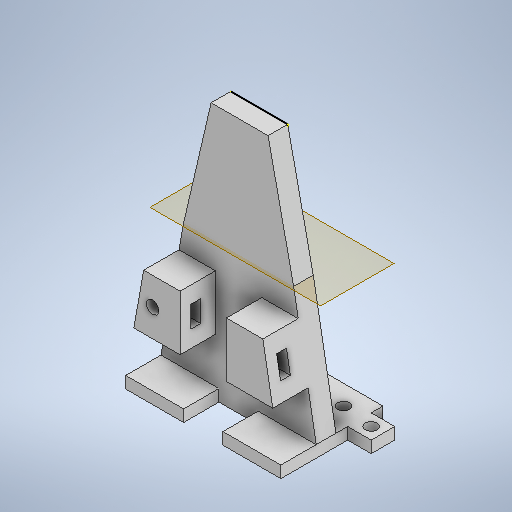
# Autodesk Inventor part: plate
Saved by Autodesk Inventor 2025 (Build 290162000, 162)
## iProperties
Created: 2025-06-05
Part Number: plate
Material: Generic
Document SubType Name: Modeling
Designer: omiye
Density: 1 g/cm^3
Appearance: Default
Author: omiye
Autodesk Inventor part; units mm, degrees
ref_plane "YZ Plane" through (0, 0, 0) normal (1, 0, 0) x (0, 1, 0)
ref_plane "XZ Plane" through (0, 0, 0) normal (0, 1, 0) x (-1, 0, 0)
ref_plane "XY Plane" through (0, 0, 0) normal (0, 0, 1) x (1, 0, 0)
sketch "Sketch1" plane through (0, 0, 0) normal (0, 1, 0) x (-1, 0, 0)
  line L0 (-50, 15) -> (50, 15)
  line L1 (50, 15) -> (50, -15)
  line L2 (50, -15) -> (-50, -15)
  line L3 (-50, -15) -> (-50, 15)
  line L4 (-50, 15) -> (50, -15) construction
  line L5 (50, 15) -> (-50, -15) construction
  point P0 (0, 0)
  dimension "d0" = 100
  dimension "d1" = 30
  constraints: 12 end point, 2 midpoint, 2 parallel, 1 horizontal, 1 perpendicular
  measures "d0" distance of L1.end L2.end
  measures "d1" distance of L0.end L1.end
extrude "Extrusion1" add sketch "Sketch1" along normal blind 3
sketch "Sketch2" plane through (0, 3, 0) normal (0, 1, 0) x (1, 0, 0)
  line L0 (25, -5) -> (-25, -5)
  line L1 (-25, -5) -> (-25, 5)
  line L2 (-25, 5) -> (25, 5)
  line L3 (25, 5) -> (25, -5)
  line L4 (25, -5) -> (-25, 5) construction
  line L5 (-25, -5) -> (25, 5) construction
  line L6 (50, 15) -> (-50, 15) projected
  line L7 (50, -15) -> (-50, -15)
  line L8 (-50, -15) -> (-50, 15)
  line L9 (-50, 15) -> (50, 15)
  line L10 (50, 15) -> (50, -15)
  line L11 (50, -15) -> (-50, 15) construction
  line L12 (-50, -15) -> (50, 15) construction
  point P0 (0, 0)
  dimension "d4" = 50
  dimension "d5" = 10
  constraints: 24 end point, 4 midpoint, 4 parallel, 2 horizontal, 2 perpendicular
  measures "d4" distance of L1.end L2.end
  measures "d5" distance of L0.end L1.end
extrude "Extrusion2" cut sketch "Sketch2" against normal blind 3
sketch "Sketch3" plane through (0, 0, 0) normal (0, -1, 0) x (1, 0, 0)
  line L0 (0, 0) -> (5, 0)
  line L1 (5, 0) -> (-5, 0)
  circle A0 centre (-5, 0) radius 1.1
  circle A1 centre (5, 0) radius 1.1
  line L2 (5, 0) -> (14.75, 0)
  line L3 (-5, 0) -> (-14.75, 0)
  circle A2 centre (14.75, 0) radius 1.1
  circle A3 centre (-14.75, 0) radius 1.1
  dimension "d8" = 5
  dimension "d9" = 10
  dimension "d10" = 2.2
  dimension "d11" = 2.2
  dimension "d12" = 9.75
  dimension "d13" = 9.75
  dimension "d14" = 2.2
  dimension "d15" = 2.2
  constraints: 8 end point, 4 centre point, 4 coincident, 2 horizontal, 2 point on line
  measures "d8" distance of L0.start L0.end
  measures "d9" distance of L0.end L1.end
  measures "d10" diameter of A0
  measures "d11" diameter of A1
  measures "d12" distance of L2.start L2.end
  measures "d13" distance of L3.start L3.end
  measures "d14" diameter of A2
  measures "d15" diameter of A3
extrude "Extrusion3" cut sketch "Sketch3" against normal blind 3.95
sketch "Sketch4" plane through (0, 3, 0) normal (0, 1, 0) x (1, 0, 0)
  circle A0 centre (-14.75, 0) radius 1.1 projected
  line L0 (-14.75, 0) -> (-19.75, 0)
  line L1 (-19.75, 0) -> (-19.75, 5)
  line L2 (25, 5) -> (-25, 5) projected
  line L3 (-19.75, 0) -> (-19.75, -5)
  line L4 (-25, -5) -> (25, -5) projected
  circle A1 centre (14.75, 0) radius 1.1 projected
  line L5 (14.75, 0) -> (19.75, 0)
  line L6 (19.75, 0) -> (19.75, 5.4669)
  line L7 (19.75, 5.4669) -> (19.75, -5)
  line L8 (-25, 5) -> (-19.75, 5)
  line L9 (-19.75, 5) -> (-19.75, -5)
  line L10 (-19.75, -5) -> (-25, -5)
  line L11 (-25, -5) -> (-25, 5)
  line L12 (19.75, -5) -> (25, -5)
  line L13 (25, -5) -> (25, 5)
  line L14 (25, 5) -> (19.75, 5)
  line L15 (19.75, 5) -> (19.75, -5)
  point P0 (0, 0)
  dimension "d18" = 5
  dimension "d19" = 5
  constraints: 28 end point, 5 point on line, 4 parallel, 4 perpendicular, 3 horizontal
  measures "d18" distance of L0.start L0.end
  measures "d19" distance of L5.start L5.end
extrude "Extrusion4" cut sketch "Sketch4" against normal blind 3.95 contours L3 L4 L11 L2 L1 | L2 L13 L4 L7 L6
sketch "Sketch5" plane through (0, 3, 0) normal (0, 1, 0) x (1, 0, 0)
  circle A0 centre (-14.75, 0) radius 1.1 projected
  line L0 (-14.75, 0) -> (-14.75, -12)
  line L1 (-19.75, -5) -> (19.75, -5) projected
  line L2 (-14.75, 0) -> (-2.75, 0) construction
  line L3 (-14.75, -12) -> (14.75, -12)
  circle A1 centre (14.75, 0) radius 1.1 projected
  line L4 (14.75, -12) -> (14.75, 0)
  line L5 (14.75, 0) -> (-14.75, 0)
  line L6 (-14.75, -12) -> (14.75, -12)
  line L7 (14.75, -12) -> (14.75, -10)
  line L8 (14.75, -10) -> (-14.75, -10)
  line L9 (-14.75, -10) -> (-14.75, -12)
  line L10 (2.5, -24) -> (-2.5, -24)
  line L11 (-2.5, -24) -> (-2.5, 0)
  line L12 (-2.5, 0) -> (2.5, 0)
  line L13 (2.5, 0) -> (2.5, -24)
  line L14 (2.5, -24) -> (-2.5, 0) construction
  line L15 (-2.5, -24) -> (2.5, 0) construction
  line L16 (-14.75, -12) -> (-19.75, -12)
  line L17 (-19.75, -12) -> (-19.75, -5)
  line L18 (-19.75, -5) -> (-14.75, -5)
  line L19 (-14.75, -5) -> (-14.75, -12)
  line L20 (14.75, -12) -> (19.75, -12)
  line L21 (19.75, -12) -> (19.75, -5)
  line L22 (19.75, -5) -> (14.75, -5)
  line L23 (14.75, -5) -> (14.75, -12)
  point P0 (0, 0)
  point P1 (0, -12)
  point P2 (2.5, -5)
  point P3 (2.5, -10)
  point P4 (-2.5, -10)
  point P5 (-2.5, -5)
  dimension "d22" = 12
  dimension "d23" = 90
  dimension "d24" = 2
  dimension "d25" = 5
  constraints: 46 end point, 9 perpendicular, 8 parallel, 4 horizontal, 3 midpoint, 1 point on line
  measures "d22" distance of L0.start L0.end
  measures "d23" angle of L0 L2
  measures "d24" distance of L7.end L6.end
  measures "d25" distance of L10.start L10.end
extrude "Extrusion5" add sketch "Sketch5" against normal up to surface (3 mm away) contours L1 L11 L8 L0 | L0 L16 L17 L1 | L8 L11 L3 L0 | L1 L4 L8 L13 | L8 L13 L3 L11 | L1 L21 L20 L4 | L8 L4 L3 L13
sketch "Sketch6" plane through (0, 3, 0) normal (0, 1, 0) x (1, 0, 0)
  line L0 (-19.75, -12) -> (-19.75, 5) projected
  line L1 (19.75, 5) -> (19.75, -12) projected
  line L2 (-19.75, -12) -> (19.75, -12)
  line L3 (19.75, -12) -> (19.75, -10)
  line L4 (19.75, -10) -> (-19.75, -10)
  line L5 (-19.75, -10) -> (-19.75, -12)
  point P0 (0, 0)
  dimension "d28" = 2
  constraints: 8 end point, 2 parallel, 1 horizontal, 1 perpendicular, 1 point on line
  measures "d28" distance of L3.end L2.end
ref_plane "Work Plane2" through (0, 35, 0) normal (0, 1, 0) x (1, 0, 0)
sketch "Sketch10" plane through (0, 35, 0) normal (0, 1, 0) x (1, 0, 0)
  line L0 (-19.75, -12) -> (19.75, -12) projected
  line L1 (0, -12) -> (-14, -12)
  line L2 (-14, -12) -> (14, -12)
  line L3 (14, -12) -> (14, -10)
  line L4 (14, -10) -> (-14, -10)
  line L5 (-14, -10) -> (-14, -12)
  point P0 (0, 0)
  dimension "d43" = 14
  dimension "d44" = 28
  dimension "d45" = 2
  constraints: 10 end point, 2 perpendicular, 2 point on line, 1 midpoint, 1 parallel
  measures "d43" distance of L1.start L1.end
  measures "d44" distance of L1.end L2.end
  measures "d45" distance of L2.end L3.end
loft "Loft2" add profiles "Sketch10", "Sketch6"
sketch "Sketch11" plane through (-14, 35, 12) normal (0, 1, 0) x (1, 0, 0)
  line L0 (33.75, 0) -> (-5.75, 0) projected
  line L1 (14, 0) -> (7, 0)
  line L2 (7, 0) -> (21, 0)
  line L3 (28, 2) -> (0, 2) projected
  line L4 (7, 0) -> (21.5, 0)
  line L5 (21.5, 0) -> (21.5, 2)
  line L6 (21.5, 2) -> (7, 2)
  line L7 (7, 2) -> (7, 0)
  point P0 (14, 12)
  point P1 (7, 2)
  point P2 (21.5, 0)
  dimension "d50" = 7
  dimension "d51" = 14
  constraints: 12 end point, 3 point on line, 2 parallel, 1 horizontal, 1 midpoint, 1 perpendicular
  measures "d50" distance of L1.start L1.end
  measures "d51" distance of L1.end L2.end
extrude "Extrusion7" add sketch "Sketch11" along normal blind 30
sketch "Sketch12" plane through (2.5, 0, 10) normal (0, 0, -1) x (-1, 0, 0)
  line L0 (2.5, 35) -> (2.5, 3)
  line L1 (5, 3) -> (0, 3) projected
  circle A0 centre (2.5, 19) radius 12.35
  point P0 (2.5, 0)
  dimension "d54" = 24.7
  constraints: 2 end point, 2 midpoint, 1 centre point
  measures "d54" diameter of A0
sketch "Sketch13" plane through (2.5, 0, 10) normal (0, 0, -1) x (-1, 0, 0)
  line L0 (16.5, 35) -> (9.5, 35) projected
  line L1 (16.5, 35) -> (9.5, 35)
  line L2 (-5, 65) -> (9.5, 65) projected
  line L3 (9.5, 35) -> (9.5, 65)
  line L4 (-5, 35) -> (-5, 65) projected
  line L5 (9.5, 65) -> (-5, 65)
  line L6 (-5, 65) -> (-5, 35)
  line L7 (-11.5, 35) -> (-5, 35) projected
  line L8 (-5, 35) -> (-11.5, 35)
  line L9 (-17.25, 3) -> (-17.25, 0) projected
  line L10 (-11.5, 35) -> (-17.25, 3)
  line L11 (16.5, 35) -> (22.25, 3) projected
  line L12 (-17.25, 3) -> (22.25, 3)
  line L13 (22.25, 3) -> (16.5, 35)
  circle A0 centre (2.5, 19) radius 12.35
  line L14 (9.5, 35) -> (-5, 35)
  point P0 (2.5, 0)
  dimension "d55" = 24.7
  constraints: 18 end point, 3 perpendicular, 2 collinear, 2 horizontal, 1 centre point, 1 parallel
  measures "d55" diameter of A0
extrude "Extrusion8" add sketch "Sketch13" along normal blind 3
extrude "Extrusion9" cut sketch "Sketch12" against normal blind 0.5
sketch "Sketch14" plane through (-2.5, 3, 5) normal (0, 0, 1) x (1, 0, 0)
  line L0 (0, 0) -> (5, 0) projected
  line L1 (0, 0) -> (0, -3) projected
  line L2 (5, 0) -> (0, 0)
  line L3 (0, 0) -> (0, -3)
  line L4 (0, -3) -> (5, -3)
  line L5 (5, -3) -> (5, 0)
  point P0 (2.5, -3)
  constraints: 8 end point, 2 parallel, 1 horizontal, 1 perpendicular
extrude "Extrusion10" cut sketch "Sketch14" against normal blind 2.5
sketch "Sketch15" plane through (-19.75, 0, 12) normal (0, 0, 1) x (1, 0, 0)
  line L0 (0, 0) -> (0, 3) projected
  line L1 (0, 0) -> (39.5, 0) projected
  line L2 (0, 3) -> (39.5, 3)
  line L3 (39.5, 3) -> (39.5, 0)
  line L4 (39.5, 0) -> (0, 0)
  line L5 (0, 0) -> (0, 3)
  point P0 (19.75, 0)
  constraints: 8 end point, 2 parallel, 1 horizontal, 1 perpendicular
extrude "Extrusion11" add sketch "Sketch15" along normal blind 9
sketch "Sketch16" plane through (-7, 65, 12) normal (0, 0, 1) x (1, 0, 0)
  line L0 (-12.75, -62) -> (26.75, -62) projected
  line L1 (7, -62) -> (7, -50.5)
  line L2 (7, -50.5) -> (1.1, -50.5)
  line L3 (1.1, -50.5) -> (7, -50.5)
  line L4 (7, -50.5) -> (12.9, -50.5)
  line L5 (12.9, -50.5) -> (22.9, -50.5)
  line L6 (22.9, -50.5) -> (1.1, -50.5)
  line L7 (1.1, -50.5) -> (-8.9, -50.5)
  line L8 (-8.9, -50.5) -> (-8.9, -36.5)
  line L9 (-8.9, -36.5) -> (1.1, -36.5)
  line L10 (1.1, -36.5) -> (1.1, -50.5)
  line L11 (12.9, -50.5) -> (12.9, -36.5)
  line L12 (12.9, -36.5) -> (22.9, -36.5)
  line L13 (22.9, -36.5) -> (22.9, -50.5)
  line L14 (1.1, -50.5) -> (-1.9, -50.5)
  line L15 (-1.9, -50.5) -> (-1.9, -36.5)
  line L16 (-1.9, -36.5) -> (1.1, -36.5)
  line L17 (1.1, -36.5) -> (1.1, -50.5)
  line L18 (12.9, -50.5) -> (15.9, -50.5)
  line L19 (15.9, -50.5) -> (15.9, -36.5)
  line L20 (15.9, -36.5) -> (12.9, -36.5)
  line L21 (12.9, -36.5) -> (12.9, -50.5)
  point P0 (7, -65)
  dimension "d64" = 11.5
  dimension "d65" = 5.9
  dimension "d66" = 5.9
  dimension "d67" = 10
  dimension "d68" = 10
  dimension "d69" = 14
  dimension "d70" = 3
  dimension "d71" = 3
  constraints: 42 end point, 5 parallel, 4 horizontal, 4 perpendicular, 4 point on line, 4 vertical, 2 collinear, 1 midpoint
  measures "d64" distance of L1.start L1.end
  measures "d65" distance of L1.end L2.end
  measures "d66" distance of L1.end L4.end
  measures "d67" distance of L4.end L5.end
  measures "d68" distance of L2.end L7.end
  measures "d69" distance of L7.end L8.end
  measures "d70" distance of L15.end L16.end
  measures "d71" distance of L20.end L19.end
extrude "Extrusion12" add sketch "Sketch16" along normal up to surface (9 mm away) contours L11 L12 L19 L5 | L7 L15 L9 L10
sketch "Sketch17" plane through (-8.9, 14.5, 21) normal (0, 0, 1) x (1, 0, 0)
  line L0 (0, 14) -> (3, 14) projected
  line L1 (0, 14) -> (-8, 14)
  line L2 (-8, 14) -> (-8, 0)
  line L3 (-8, 0) -> (0, 0)
  line L4 (0, 0) -> (0, 14)
  line L5 (17.8, 14) -> (17.8, 0) projected
  line L6 (17.8, 14) -> (25.8, 14)
  line L7 (25.8, 14) -> (25.8, 0)
  line L8 (25.8, 0) -> (17.8, 0)
  line L9 (17.8, 0) -> (17.8, 14)
  line L10 (-8, 7) -> (-4, 7)
  circle A0 centre (-4, 7) radius 1.6
  line L11 (25.8, 0) -> (21.8, 0)
  line L12 (25.8, 7) -> (21.8, 7)
  circle A1 centre (21.8, 7) radius 1.6
  point P0 (8.9, -14.5)
  dimension "d74" = 8
  dimension "d75" = 8
  dimension "d76" = 3.2
  dimension "d77" = 3.2
  constraints: 22 end point, 4 horizontal, 4 parallel, 3 midpoint, 2 centre point, 2 coincident, 2 perpendicular, 1 point on line
  measures "d74" distance of L3.end L2.end
  measures "d75" distance of L7.end L8.end
  measures "d76" diameter of A0
  measures "d77" diameter of A1
extrude "Extrusion13" add sketch "Sketch17" against normal blind 3
sketch "Sketch18" plane through (-19.75, 0, -5) normal (-1, 0, 0) x (0, 0, 1)
  line L0 (0, 0) -> (0, 3) projected
  line L1 (12, 35) -> (12, 3) projected
  line L2 (0, 0) -> (12, 0)
  line L3 (12, 0) -> (12, 3)
  line L4 (12, 3) -> (0, 3)
  line L5 (0, 3) -> (0, 0)
  line L6 (12, 3) -> (0, 3) projected
  line L7 (5, 0) -> (9, 0)
  line L8 (9, 0) -> (9, 3)
  line L9 (9, 3) -> (5, 3)
  line L10 (5, 3) -> (5, 0)
  line L11 (5, 0) -> (3, 0)
  line L12 (3, 0) -> (3, 3)
  line L13 (3, 3) -> (5, 3)
  line L14 (5, 3) -> (5, 0)
  point P0 (3, 3)
  point P1 (3, 0)
  dimension "d80" = 4
  dimension "d81" = 2
  constraints: 24 end point, 6 parallel, 3 horizontal, 3 perpendicular, 2 point on line
  measures "d80" distance of L9.end L8.end
  measures "d81" distance of L12.end L13.end
extrude "Extrusion14" add sketch "Sketch18" along normal blind 6 contours L12 L4 L10 L2 | L10 L4 L8 L2
sketch "Sketch19" plane through (19.75, 0, -5) normal (1, 0, 0) x (0, 0, -1)
  line L0 (-9, 3) -> (-3, 3) projected
  line L1 (-5, 0) -> (-9, 0)
  line L2 (-9, 0) -> (-9, 3)
  line L3 (-9, 3) -> (-5, 3)
  line L4 (-5, 3) -> (-5, 0)
  line L5 (-5, 0) -> (-3, 0)
  line L6 (-3, 0) -> (-3, 3)
  line L7 (-3, 3) -> (-5, 3)
  line L8 (-5, 3) -> (-5, 0)
  dimension "d84" = 4
  dimension "d85" = 2
  constraints: 16 end point, 4 parallel, 2 horizontal, 2 perpendicular, 1 point on line
  measures "d84" distance of L0.start L3.end
  measures "d85" distance of L7.end L6.end
extrude "Extrusion15" add sketch "Sketch19" along normal blind 6
sketch "Sketch20" plane through (0, 3, 0) normal (0, 1, 0) x (1, 0, 0)
  line L0 (25.75, -4) -> (25.75, 2) projected
  line L1 (25.75, -1) -> (22.75, -1)
  circle A0 centre (22.75, -1) radius 1.525
  line L2 (-25.75, -4) -> (-25.75, 2) projected
  line L3 (-25.75, -1) -> (-22.75, -1)
  circle A1 centre (-22.75, -1) radius 1.525
  point P0 (0, 0)
  dimension "d88" = 3
  dimension "d89" = 3.05
  dimension "d90" = 3
  dimension "d91" = 3.05
  constraints: 4 end point, 2 centre point, 2 coincident, 2 horizontal, 2 midpoint
  measures "d88" distance of L1.start L1.end
  measures "d89" diameter of A0
  measures "d90" distance of L3.start L3.end
  measures "d91" diameter of A1
extrude "Extrusion16" cut sketch "Sketch20" against normal blind 6
sketch "Sketch21" plane through (2.5, 0, 7) normal (0, 0, -1) x (-1, 0, 0)
  line L0 (9.5, 35) -> (9.5, 65) projected
  line L1 (-5, 35) -> (-5, 65) projected
  line L2 (9.5, 65) -> (-5, 65)
  line L3 (-5, 65) -> (-5, 35)
  line L4 (-5, 35) -> (9.5, 35)
  line L5 (9.5, 35) -> (9.5, 65)
  point P0 (2.5, 0)
  constraints: 8 end point, 2 parallel, 1 horizontal, 1 perpendicular
sketch "Sketch22" plane through (2.5, 0, 7) normal (0, 0, -1) x (-1, 0, 0)
  line L0 (16.5, 35) -> (9.5, 35) projected
  line L1 (9.5, 35) -> (9.5, 65) projected
  line L2 (16.5, 35) -> (9.5, 65)
  line L3 (-5, 35) -> (-5, 65) projected
  line L4 (9.5, 65) -> (-5, 65)
  line L5 (-11.5, 35) -> (-17.25, 3) projected
  line L6 (-5, 65) -> (-11.5, 35)
  line L7 (-5, 35) -> (-11.5, 35) projected
  line L8 (-5, 35) -> (-11.5, 35)
  point P0 (2.5, 0)
  constraints: 8 end point, 1 collinear, 1 perpendicular
extrude "Extrusion17" add sketch "Sketch22" against normal up to surface (5 mm away)
sketch "Sketch23" plane through (0, 3, 0) normal (0, 1, 0) x (1, 0, 0)
  circle A0 centre (-14.75, 0) radius 1.1 projected
  circle A1 centre (-14.75, 0) radius 1.5
  circle A2 centre (-5, 0) radius 1.1 projected
  circle A3 centre (-5, 0) radius 1.5
  circle A4 centre (5, 0) radius 1.1 projected
  circle A5 centre (5, 0) radius 1.5
  circle A6 centre (14.75, 0) radius 1.1 projected
  circle A7 centre (14.75, 0) radius 1.5
  point P0 (0, 0)
  dimension "d96" = 3
  dimension "d97" = 3
  dimension "d98" = 3
  dimension "d99" = 3
  constraints: 4 centre point, 4 coincident
  measures "d96" diameter of A1
  measures "d97" diameter of A3
  measures "d98" diameter of A5
  measures "d99" diameter of A7
extrude "Extrusion18" cut sketch "Sketch23" against normal blind 10 contours A0 | A1 | A3 | A4 | A5 | A6 | A7
sketch "Sketch24" plane through (-19.75, 3, 12) normal (0, 0, 1) x (1, 0, 0)
  line L0 (10.85, 11.5) -> (2.85, 11.5) projected
  line L1 (2.85, 11.5) -> (2.0664, 11.5)
  line L2 (0, 0) -> (5.75, 32) projected
  line L3 (2.0664, 11.5) -> (4.582, 25.5)
  line L4 (10.85, 25.5) -> (13.85, 25.5) projected
  line L5 (13.85, 25.5) -> (4.582, 25.5)
  line L6 (13.85, 25.5) -> (13.85, 11.5)
  line L7 (13.85, 11.5) -> (2.0664, 11.5)
  circle A0 centre (6.85, 18.5) radius 1.6 projected
  circle A1 centre (6.85, 18.5) radius 1.6
  line L8 (13.85, 11.5) -> (13.85, 25.5)
  line L9 (33.75, 32) -> (39.5, 0) projected
  line L10 (34.918, 25.5) -> (37.4336, 11.5)
  line L11 (25.65, 11.5) -> (36.65, 11.5) projected
  line L12 (25.65, 11.5) -> (37.4336, 11.5)
  line L13 (25.65, 25.5) -> (28.65, 25.5) projected
  line L14 (25.65, 11.5) -> (25.65, 25.5)
  line L15 (25.65, 25.5) -> (34.918, 25.5)
  circle A2 centre (32.65, 18.5) radius 1.6 projected
  circle A3 centre (32.65, 18.5) radius 1.6
  point P0 (19.75, -3)
  dimension "d102" = 3.2
  constraints: 20 end point, 4 point on line, 3 collinear, 3 perpendicular, 2 centre point, 2 coincident, 1 horizontal, 1 vertical
  measures "d102" diameter of A1
extrude "Extrusion19" add sketch "Sketch24" along normal up to surface (9 mm away) contours L0 L1 L2 L5 L4 L6 L7 | L9 L12 L11 L14 L13 L15 | A2
sketch "Sketch25" plane through (-17.6836, 14.5, 21) normal (0, 0, 1) x (1, 0, 0)
  line L0 (0.7836, 14) -> (2.5156, 14) projected
  line L1 (2.5156, 14) -> (0.7836, 4.3609) projected
  line L2 (2.5156, 14) -> (0.7836, 4.3609)
  line L3 (0.7836, 4.3609) -> (0.7836, 14) projected
  line L4 (0.7836, 4.3609) -> (0.7836, 14)
  line L5 (0.7836, 14) -> (2.5156, 14)
  line L6 (34.5836, 4.3609) -> (32.8516, 14) projected
  line L7 (32.8516, 14) -> (34.5836, 4.3609)
  line L8 (34.5836, 4.3609) -> (34.5836, 14) projected
  line L9 (34.5836, 4.3609) -> (34.5836, 14)
  line L10 (34.5836, 14) -> (32.8516, 14)
  point P0 (17.6836, -14.5)
  constraints: 12 end point, 4 collinear, 2 perpendicular
extrude "Extrusion20" cut sketch "Sketch25" against normal blind 10
sketch "Sketch26" plane through (-19.75, 3, 7) normal (-1, 0, 0) x (0, 0, 1)
  line L0 (14, 11.5) -> (14, 25.5) projected
  line L1 (14, 18.5) -> (10, 18.5)
  line L2 (11.25, 15.75) -> (11.25, 21.25)
  line L3 (11.25, 21.25) -> (8.75, 21.25)
  line L4 (8.75, 21.25) -> (8.75, 15.75)
  line L5 (8.75, 15.75) -> (11.25, 15.75)
  line L6 (11.25, 15.75) -> (8.75, 21.25) construction
  line L7 (11.25, 21.25) -> (8.75, 15.75) construction
  line L8 (5, 16.9) -> (14, 16.9) projected
  line L9 (11.25, 15.75) -> (16.75, 15.75) construction
  point P0 (-7, -3)
  dimension "d107" = 4
  dimension "d108" = 5.5
  dimension "d109" = 90
  dimension "d110" = 2.5
  constraints: 16 end point, 3 midpoint, 3 perpendicular, 2 horizontal, 2 parallel
  measures "d107" distance of L1.start L1.end
  measures "d108" distance of L2.start L2.end
  measures "d109" angle of L9 L2
  measures "d110" distance of L3.end L2.end
extrude "Extrusion21" cut sketch "Sketch26" against normal blind 49 contours L8 L4 L3 L2 | L2 L5 L4 L8
sketch "Sketch27" plane through (0, 0, 0) normal (0, -1, 0) x (1, 0, 0)
  line L0 (-5, 30) -> (5, 30)
  line L1 (5, 30) -> (5, 12)
  line L2 (5, 12) -> (-5, 12)
  line L3 (-5, 12) -> (-5, 30)
  line L4 (-19.75, 21) -> (19.75, 21) projected
  line L5 (-5, 30) -> (5, 12) construction
  line L6 (5, 30) -> (-5, 12) construction
  line L7 (5, 21) -> (-5, 21)
  point P0 (0, 0)
  point P1 (0, 21)
  dimension "d113" = 10
  constraints: 14 end point, 5 midpoint, 2 parallel, 2 point on line, 1 perpendicular
  measures "d113" distance of L0.start L0.end
extrude "Extrusion22" cut sketch "Sketch27" against normal blind 3.5 contours L4 L1 L2 L3
body "Solid1"
